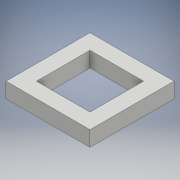
# Autodesk Inventor part: Key Cap Hole Test
Saved by Autodesk Inventor 2018 (Build 220112000, 112)
## iProperties
Created: 2018-05-25
Part Number: Key Cap Hole Test
Material: Generic
Document SubType Name: Modeling
Designer: mtsti
Density: 1 g/cm^3
Appearance: Default
Author: mtsti
Autodesk Inventor part; units mm, degrees
ref_plane "YZ Plane" through (0, 0, 0) normal (1, 0, 0) x (0, 1, 0)
ref_plane "XZ Plane" through (0, 0, 0) normal (0, 1, 0) x (-1, 0, 0)
ref_plane "XY Plane" through (0, 0, 0) normal (0, 0, 1) x (1, 0, 0)
sketch "Sketch1" plane through (0, 0, 0) normal (0, 0, 1) x (1, 0, 0)
  line L0 (0, 0) -> (14, 0)
  line L1 (14, 0) -> (14, 14)
  line L2 (14, 14) -> (0, 14)
  line L3 (0, 14) -> (0, 0)
  line L4 (-4, -4) -> (18, -4)
  line L5 (18, -4) -> (18, 18)
  line L6 (18, 18) -> (-4, 18)
  line L7 (-4, 18) -> (-4, -4)
  dimension "d0" = 14
  dimension "d1" = 14
  dimension "d2" = 4
  dimension "d3" = 4
  dimension "d4" = 4
  dimension "d5" = 4
  constraints: 16 end point, 4 parallel, 2 horizontal, 2 perpendicular
  measures "d0" distance of L2.end L1.end
  measures "d1" distance of L1.end L0.end
  measures "d2" distance between parallel lines of L3 L7
  measures "d3" distance between parallel lines of L4 L0
  measures "d4" distance between parallel lines of L6 L2
  measures "d5" distance between parallel lines of L1 L5
extrude "Extrusion1" add sketch "Sketch1" along normal blind 4
body "Solid1"
